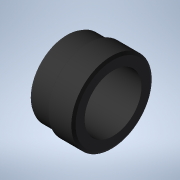
# Autodesk Inventor part: SCHUNK-9951430 Zentrierhuelse PGN-plus
Saved by Autodesk Inventor 2021 (Build 250183000, 183)
## iProperties
Created: 2025-07-30
Part Number: SCHUNK-9951430 Zentrierhuelse PGN-plus
Material: Generic
Catalog Web Link: www.cadenas.de
Description: Zentrierhuelse mit Absatz fuer Praezisionsausfuehrung-Zentrierhuelse mit Absatz
Vendor: SCHUNK
Document SubType Name: Modeling
Designer: psAdmin
Manufacturer: SCHUNK
Mass: 0.666517 g
Surface Area: 8.32594 cm^2
Volume: 0.666517 cm^3
Density: 1 g/cm^3
Appearance: PSOLRGB-175-175-175
Category: PARTsolutions
Company: SCHUNK
Title: SCHUNK-9951430 Zentrierhuelse PGN-plus
Author: Cadenas PARTsolutions
Comments: Zentrierhuelse mit Absatz
PSOL_IDENT_0: {$CADENAS_DATA/23d-libs/schunk/greifsysteme/greifmodule/greifmodule_pneumatisch/2_finger_parallelgre
PSOL_IDENT_1: ifer/2_finger_universalgreifer/pgn_plus/pgnplus_zhu_mit_abs.prj},263 {VTYP=3D},{NB=SCHUNK-9951430 Ze
PSOL_IDENT_2: ntrierhuelse PGN-plus},{LINA=SCHUNK-9951430 Zentrierhuelse PGN-plus},{NN=Zentrierhuelse mit Absatz f
PSOL_IDENT_3: uer Praezisionsausfuehrung},{DATE=18.12.2024 09:59:26},{GEOMDATE=15.04.2020 08:38:35},{VERSION=},{LI
PSOL_IDENT_4: NEID=60},{WBVAR=},{WBNUMERIC=}  {NB=SCHUNK-9951430 Zentrierhuelse PGN-plus},{LINA=SCHUNK-9951430 Zen
PSOL_IDENT_5: trierhuelse PGN-plus},{KT=DUMMY},{IDNR=9951430},{TYP=PGN-plus},{TYPZHU=2.000},{ZH=6.000},{D1=15.000}
PSOL_IDENT_6: ,{L1=8.600},{D2=0.000},{L2=0.000},{D3=14.000},{L3=3.850},{D4=0.000},{L4=0.000},{FL=0.500},{D5=10.600
PSOL_IDENT_7: },{CNSCTN=73182900}
NB: SCHUNK-9951430 Zentrierhuelse PGN-plus
NN: Zentrierhuelse mit Absatz fuer Praezisionsausfuehrung
NT: Zentrierhuelse mit Absatz
NBSYN: SCHUNK-$IDNR. Zentrierhuelse $TYP.
LINA: SCHUNK-9951430 Zentrierhuelse PGN-plus
CATALOG: SCHUNK
IDNR: 9951430
TYP: PGN-plus
CNSCTN: 73182900
SUPPLIER: SCHUNK
ARTICLENO: SCHUNK-9951430 Zentrierhuelse PGN-plus
BOMINFO: SCHUNK-9951430 Zentrierhuelse PGN-plus
CREATOR: CADENAS GmbH
Autodesk Inventor part; units mm, degrees
sketch "Sketch_1" plane through (0, 0, 0) normal (0, 1, 0) x (-1, 0, 0)
  line L0 (-8.6, 0) -> (0, 0)
  line L1 (0, 0) -> (0, -7.5)
  line L2 (0, -7.5) -> (-8.3113, -7.5)
  line L3 (-8.3113, -7.5) -> (-8.6, -7)
  line L4 (-8.6, -7) -> (-8.6, 0)
  line L5 (-8.6, 0) -> (0, 0)
  constraints: 12 end point
revolve "Revolution1" add sketch "Sketch_1" angle 360 about axis through (8.6, 0, 0) along (1, 0, 0)
sketch "Sketch_2" plane through (0, 0, 0) normal (0, 1, 0) x (-1, 0, 0)
  line L0 (-50, 0) -> (50, 0)
  line L1 (0, -6.75) -> (-0.433, -7)
  line L2 (-0.433, -7) -> (-3.85, -7)
  line L3 (-3.85, -7) -> (-3.85, -7.5)
  line L4 (-3.85, -7.5) -> (0, -7.5)
  line L5 (0, -7.5) -> (0, -6.75)
  constraints: 12 end point
revolve "Revolution2" cut sketch "Sketch_2" angle 360 about axis through (50, 0, 0) along (1, 0, 0)
sketch "Sketch_3" plane through (0, 0, 0) normal (0, 1, 0) x (-1, 0, 0)
  line L0 (-50, 0) -> (50, 0)
  line L1 (-3.85, -7.5) -> (-3.85, -7.3)
  line L2 (-3.85, -7.3) -> (-4.05, -7.5)
  line L3 (-4.05, -7.5) -> (-3.85, -7.5)
  constraints: 8 end point
revolve "Revolution3" cut sketch "Sketch_3" angle 360 about axis through (50, 0, 0) along (1, 0, 0)
sketch "Sketch4" plane through (8.6, 0, 0) normal (1, 0, 0) x (0, 0, -1)
  point P0 (0, 0)
hole "Hole1" at (8.6, 0, 0) direction (-1, 0, 0) diameter 10.6 depth 8.6
ref_plane "gba_XY" through (8.6, 0, 0) normal (1, 0, 0) x (0, 0, -1)
ref_plane "gba_YZ" through (8.6, 0, 0) normal (0, 0, -1) x (0, 1, 0)
ref_plane "gba_ZX" through (8.6, 0, 0) normal (0, 1, 0) x (1, 0, 0)
body "Solid1"
